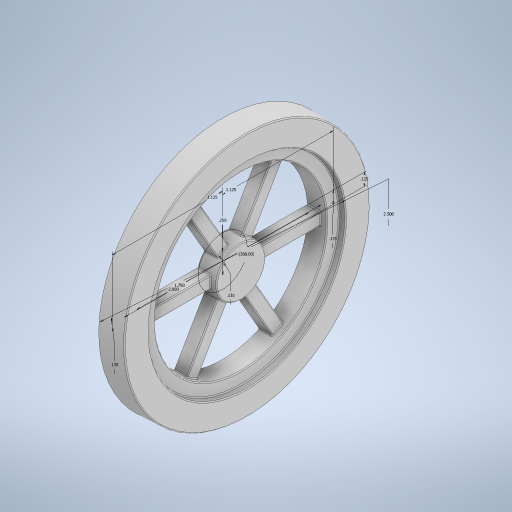
# Autodesk Inventor part: Flywheel Cast Image
Saved by Autodesk Inventor 2023 (Build 270158000, 158)
## iProperties
Created: 2022-12-28
Part Number: Flywheel Cast Image
Material: Generic
Document SubType Name: Modeling
Designer: tgr41
Density: 1 g/cm^3
Appearance: Default
Author: tgr41
Autodesk Inventor part; units mm, degrees
ref_plane "YZ Plane" through (0, 0, 0) normal (1, 0, 0) x (0, 1, 0)
ref_plane "XZ Plane" through (0, 0, 0) normal (0, 1, 0) x (-1, 0, 0)
ref_plane "XY Plane" through (0, 0, 0) normal (0, 0, 1) x (1, 0, 0)
sketch "Sketch1" plane through (0, 0, 0) normal (1, 0, 0) x (0, 1, 0)
  circle A0 centre (0, 0) radius 31.75
  circle A1 centre (0, 0) radius 6.35
  line L0 (-1.5875, -6.1484) -> (-1.5875, -22.1682)
  line L1 (1.5875, -6.1484) -> (1.5875, -22.1682)
  circle A2 centre (0, 0) radius 3.175
  circle A3 centre (0, 0) radius 25.4
  circle A4 centre (0, 0) radius 22.225
  line L2 (4.5309, -4.449) -> (18.4045, -12.4589)
  line L3 (6.1184, -1.6994) -> (19.992, -9.7093)
  line L4 (6.1184, 1.6994) -> (19.992, 9.7093)
  line L5 (4.5309, 4.449) -> (18.4045, 12.4589)
  line L6 (1.5875, 6.1484) -> (1.5875, 22.1682)
  line L7 (-1.5875, 6.1484) -> (-1.5875, 22.1682)
  line L8 (-4.5309, 4.449) -> (-18.4045, 12.4589)
  line L9 (-6.1184, 1.6994) -> (-19.992, 9.7093)
  line L10 (-6.1184, -1.6994) -> (-19.992, -9.7093)
  line L11 (-4.5309, -4.449) -> (-18.4045, -12.4589)
  circle A5 centre (0, -28.575) radius 1.7145
  circle A6 centre (0, 0) radius 1.7145
  circle A7 centre (0, 28.575) radius 1.7145
  point P0 (-1.5875, 22.1682)
  point P1 (-1.5875, 6.1484)
  point P2 (19.992, -9.7093)
  dimension "d8" = 6.35
  dimension "d11" = 50.8
  dimension "d18" = 63.5
  dimension "d19" = 44.45
  dimension "d22" = 360
  dimension "d28" = 3.175
  dimension "d33" = 3.429
  dimension "d34" = 3.429
  dimension "d35" = 3.429
  dimension "d36" = 28.575
  dimension "d37" = 28.575
  constraints: 24 end point, 8 centre point, 5 point on circle, 4 coincident, 1 vertical, 37 other
  measures "d8" diameter of A2
  measures "d11" diameter of A3
  measures "d18" diameter of A0
  measures "d19" diameter of A4
  measures "d28" distance between parallel lines of L1 L0
  measures "d33" diameter of A5
  measures "d34" diameter of A6
  measures "d35" diameter of A7
  measures "d36" distance of A0.centre A7.centre
  measures "d37" distance of A0.centre A5.centre
extrude "Extrusion2" add sketch "Sketch1" along normal mid plane 12.7 contours A0 | A5 | A7
extrude "Extrusion5" add sketch "Sketch1" along normal mid plane 9.525 contours A1 | A2 | A3 | A6
extrude "Extrusion6" add sketch "Sketch1" along normal mid plane 6.35 contours A1 L5 A4 L4 | L3 A4 L2 A1 | A1 L7 A4 L6 | L1 A4 L0 A1 | A1 L9 A4 L8 | L11 A4 L10 A1
sketch "Sketch2" plane through (0, 0, 0) normal (0, 1, 0) x (-1, 0, 0)
  line L0 (6.35, 25.4) -> (6.35, -25.4) projected
  line L1 (6.35, 0) -> (-6.35, 0)
  line L2 (-6.35, -25.4) -> (-6.35, 25.4) projected
  line L3 (0, 0) -> (0, 38.961)
  line L4 (0, 38.961) -> (11.1473, 38.961)
  line L5 (11.1473, 38.961) -> (11.1473, -36.7752)
  line L6 (11.1473, -36.7752) -> (0, -36.7752)
  line L7 (0, -36.7752) -> (0, 0)
  constraints: 12 end point, 3 perpendicular, 2 midpoint, 1 collinear, 1 point on line, 1 vertical
extrude "Extrusion7" cut sketch "Sketch2" along normal mid plane 77.7875
draft "FaceDraft1" angle -2.5 pull direction (-1, 0, 0) faces at (4.2333, 31.647, -2.5548) (2.6458, -5.3658, -21.5675) (2.1167, -13.78, 9.789) (1.0583, 1.5875, 11.4883) (2.1167, 9.1554, 7.119) (1.0583, 15.3675, -7.0393) (1.0583, 1.5875, -16.8283) (2.1167, -15.3675, -7.0393) (2.1167, -9.1554, -7.119) (2.1167, 13.78, -9.789) (1.0583, 15.3675, 7.0393) (2.6458, -2.6474, -5.7718) (2.1167, -10.7429, 4.3693) (1.0583, -1.5875, 16.8283) (1.0583, -1.5875, -11.4883) (5.8208, 25.3176, -2.0439) fixed edges at (6.35, -31.75, 0) (4.7625, -22.225, 0) (3.175, -11.4677, 8.454) (3.175, 1.5875, 14.1583) (3.175, 11.4677, 8.454) (3.175, 13.0552, -5.7043) (3.175, 1.5875, -14.1583) (3.175, -13.0552, -5.7043) (3.175, -11.4677, -8.454) (3.175, 11.4677, -8.454) (3.175, 13.0552, 5.7043) (4.7625, -6.35, 0) (3.175, -13.0552, 5.7043) (3.175, -1.5875, 14.1583) (3.175, -1.5875, -14.1583) (6.35, -25.4, 0)
fillet "Fillet1" radius 0.254 53 edges at (4.7625, -22.225, 0) (3.175, -11.4686, -8.4545) (3.175, -13.0561, -5.7049) (3.175, -19.1874, -11.0778) (3.175, -19.1874, 11.0778) (3.175, -13.0561, 5.7049) (3.175, -11.4686, 8.4545) (1.5848, -18.2449, -12.447) (1.5848, -18.2449, 12.447) (3.175, -1.5875, 14.1593) (3.175, 1.5875, 14.1593) (3.175, 11.4686, 8.4545) (3.175, 13.0561, 5.7049) (3.175, 13.0561, -5.7049) (3.175, 11.4686, -8.4545) (3.175, 1.5875, -14.1593) (3.175, -1.5875, -14.1593) (4.7625, -6.35, 0) (3.175, 0, -6.4193) (1.5943, 1.6565, -6.2733) (3.175, 5.5593, -3.2097) (1.5943, 6.2611, -1.7021) (1.5943, 6.2611, 1.7021) (3.175, 5.5593, 3.2097) (1.5943, 1.6565, 6.2733) (3.175, 0, 6.4193) (1.5943, 4.6046, 4.5712) (1.5943, -4.6046, 4.5712) (3.175, -5.5593, 3.2097) (1.5848, -19.9018, -9.5771) (1.5848, -1.6569, -22.024) (3.175, 0, -22.1557) (3.175, 19.1874, -11.0778) (1.5848, 19.9018, -9.5771) (1.5943, -1.6565, 6.2733) (6.35, -31.75, 0) (1.5848, 1.6569, -22.024) (1.5848, 18.2449, -12.447) (1.5848, 18.2449, 12.447) (1.5848, 19.9018, 9.5771) (1.5848, -1.6569, 22.024) (3.175, 0, 22.1557) (3.175, 19.1874, 11.0778) (1.5848, -19.9018, 9.5771) (1.5848, 1.6569, 22.024) (1.5943, -4.6046, -4.5712) (1.5943, 4.6046, -4.5712) (1.5943, -6.2611, 1.7021) (1.5943, -6.2611, -1.7021) (1.5943, -1.6565, -6.2733) (3.175, -5.5593, -3.2097) (4.7625, -25.3307, 0) (6.35, -25.4, 0)
extrude "Extrusion8" cut sketch "Sketch1" along normal blind 3.175 contours A5 | A6 | A7
body "Solid2"
